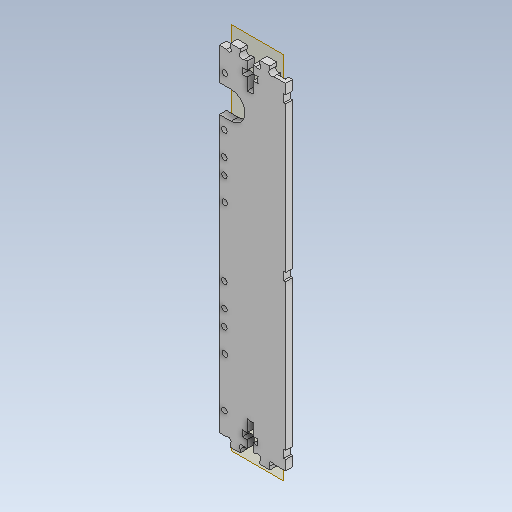
# Autodesk Inventor part: side_top
Saved by Autodesk Inventor 2020 (Build 240168000, 168)
## iProperties
Created: 2020-01-09
Part Number: side_top
Material: Generic
Document SubType Name: Modeling
Designer: erwin
Density: 1 g/cm^3
Appearance: Default
Author: erwin
Autodesk Inventor part; units mm, degrees
ref_plane "YZ Plane" through (0, 0, 0) normal (1, 0, 0) x (0, 1, 0)
ref_plane "XZ Plane" through (0, 0, 0) normal (0, 1, 0) x (-1, 0, 0)
ref_plane "XY Plane" through (0, 0, 0) normal (0, 0, 1) x (1, 0, 0)
ref_plane "Work Plane1" through (0, 0, 0) normal (0, 0, 1) x (1, 0, 0)
sketch "Sketch1" plane through (0, 0, 0) normal (0, 0, 1) x (1, 0, 0)
  line L0 (30, 0) -> (23.9528, 0) projected
  line L1 (30, 0) -> (30, -5) projected
  line L2 (23.9799, -170) -> (30, -170) projected
  line L3 (22, -171.9799) -> (22, -173.6) projected
  line L4 (22, -173.6) -> (17, -173.6) projected
  line L5 (17, -173.6) -> (17, -171.9799) projected
  line L6 (15.0201, -170) -> (13.5, -170) projected
  line L7 (13.5, -170) -> (13.5, -166) projected
  line L8 (13.5, -166) -> (16, -166) projected
  line L9 (16, -166) -> (16, -163) projected
  line L10 (16, -163) -> (13.5, -163) projected
  line L11 (13.5, -163) -> (13.5, -157) projected
  line L12 (13.5, -157) -> (10.5, -157) projected
  line L13 (10.5, -157) -> (10.5, -163) projected
  line L14 (10.5, -163) -> (8, -163) projected
  line L15 (8, -163) -> (8, -166) projected
  line L16 (8, -166) -> (10.5, -166) projected
  line L17 (10.5, -166) -> (10.5, -170) projected
  line L18 (10.5, -170) -> (8.9799, -170) projected
  line L19 (7, -171.9799) -> (7, -173.6) projected
  line L20 (7, -173.6) -> (2, -173.6) projected
  line L21 (2, -173.6) -> (2, -171.9799) projected
  line L22 (0.0201, -170) -> (-3.6, -170) projected
  line L23 (-3.6, -170) -> (-3.6, 0) projected
  line L24 (-3.6, 0) -> (0.0472, 0) projected
  line L25 (2, 1.9528) -> (2, 3.6) projected
  line L26 (2, 3.6) -> (7, 3.6) projected
  line L27 (7, 3.6) -> (7, 1.9799) projected
  line L28 (8.9799, 0) -> (10.5, 0) projected
  line L29 (10.5, 0) -> (10.5, -4) projected
  line L30 (10.5, -4) -> (8, -4) projected
  line L31 (8, -4) -> (8, -7) projected
  line L32 (8, -7) -> (10.5, -7) projected
  line L33 (10.5, -7) -> (10.5, -13) projected
  line L34 (10.5, -13) -> (13.5, -13) projected
  line L35 (13.5, -13) -> (13.5, -7) projected
  line L36 (13.5, -7) -> (16, -7) projected
  line L37 (16, -7) -> (16, -4) projected
  line L38 (16, -4) -> (13.5, -4) projected
  line L39 (13.5, -4) -> (13.5, 0) projected
  line L40 (13.5, 0) -> (15.0472, 0) projected
  line L41 (17, 1.9528) -> (17, 3.6) projected
  line L42 (17, 3.6) -> (22, 3.6) projected
  line L43 (22, 3.6) -> (22, 1.9528) projected
  line L44 (29, -165) -> (30, -165) projected
  line L45 (30, -5) -> (29, -5) projected
  line L46 (29, -5) -> (29, -9) projected
  line L47 (29, -9) -> (30, -9) projected
  line L48 (30, -9) -> (30, -83) projected
  line L49 (30, -83) -> (29, -83) projected
  line L50 (29, -83) -> (29, -87) projected
  line L51 (29, -87) -> (30, -87) projected
  line L52 (30, -87) -> (30, -161) projected
  line L53 (30, -161) -> (29, -161) projected
  line L54 (29, -161) -> (29, -165) projected
  arc A0 (17, -171.9799) -> (15.0201, -170) centre (16.0101, -170.9899) ccw projected
  arc A1 (8.9799, -170) -> (7, -171.9799) centre (7.9899, -170.9899) ccw projected
  arc A2 (2, -171.9799) -> (0.0201, -170) centre (1.0101, -170.9899) ccw projected
  arc A3 (0.0472, 0) -> (2, 1.9528) centre (1.1868, 0.8132) ccw projected
  arc A4 (7, 1.9799) -> (8.9799, 0) centre (7.9899, 0.9899) ccw projected
  arc A5 (15.0472, 0) -> (17, 1.9528) centre (16.1868, 0.8132) ccw projected
  arc A6 (22, 1.9528) -> (23.9528, 0) centre (22.8132, 0.8132) ccw projected
  line L55 (30, -165) -> (30, -170) projected
  arc A7 (23.9799, -170) -> (22, -171.9799) centre (22.9899, -170.9899) ccw projected
  circle A8 centre (-0.9899, -159.0101) radius 1.4 projected
  circle A9 centre (-0.8132, -134.0132) radius 1.4 projected
  circle A10 centre (-0.9899, -122.2101) radius 1.4 projected
  circle A11 centre (-0.9899, -114.1899) radius 1.4 projected
  circle A12 centre (-0.9899, -102.2101) radius 1.4 projected
  circle A13 centre (-0.8132, -67.6132) radius 1.4 projected
  circle A14 centre (-0.9899, -55.8101) radius 1.4 projected
  circle A15 centre (-0.9899, -47.7899) radius 1.4 projected
  circle A16 centre (-0.9899, -35.8101) radius 1.4 projected
  circle A17 centre (-0.8132, -10.8132) radius 1.4 projected
  point P0 (0, 0)
  point P1 (22, 0)
  point P2 (22, -170)
  point P3 (17, -170)
  point P4 (7, -170)
  point P5 (2, -170)
  point P6 (0, -160)
  point P7 (0, -123.2)
  point P8 (0, -113.2)
  point P9 (0, -103.2)
  point P10 (0, -56.8)
  point P11 (0, -46.8)
  point P12 (0, -36.8)
  point P13 (2, 0)
  point P14 (7, 0)
  point P15 (17, 0)
  point P16 (-1.9799, -160)
  point P17 (-1.9528, -133.2)
  point P18 (-1.9799, -123.2)
  point P19 (-1.9799, -113.2)
  point P20 (-1.9799, -103.2)
  point P21 (-1.9528, -66.8)
  point P22 (-1.9799, -56.8)
  point P23 (-1.9799, -46.8)
  point P24 (-1.9799, -36.8)
  point P25 (-1.9528, -10)
  point P26 (0, -34.8201)
  point P27 (0, -11.9528)
  point P28 (0, -54.8201)
  point P29 (0, -48.7799)
  point P30 (0, -101.2201)
  point P31 (0, -68.7528)
  point P32 (0, -121.2201)
  point P33 (0, -115.1799)
  point P34 (0, -158.0201)
  point P35 (0, -135.1528)
  constraints: 3 other
extrude "Extrusion1" add sketch "Sketch1" along normal blind 3.6
sketch "Sketch3" plane through (0, 0, 0) normal (0, 0, -1) x (-1, 0, 0)
  line L0 (-28, -170) -> (-24, -170) projected
  line L1 (-28, 0) -> (-28, -170) projected
  line L2 (-24, 0) -> (-28, 0) projected
  line L3 (-24, 0) -> (-24, -170) projected
  point P0 (0, 0)
extrude "Extrusion3" cut sketch "Sketch3" against normal blind 1.8
sketch "Sketch16" plane through (0, 0, 3.6) normal (0, 0, 1) x (1, 0, 0)
  line L0 (30, -87) -> (29, -87) projected
  line L1 (29, -87) -> (29, -83) projected
  line L2 (29, -83) -> (30, -83) projected
  line L3 (30, -83) -> (30, -9) projected
  line L4 (30, -9) -> (29, -9) projected
  line L5 (29, -9) -> (29, -5) projected
  line L6 (29, -5) -> (30, -5) projected
  line L7 (30, -5) -> (30, 0) projected
  line L8 (30, 0) -> (23.9528, 0) projected
  arc A0 (22, 1.9528) -> (23.9528, 0) centre (22.8132, 0.8132) ccw projected
  line L9 (22, 1.9528) -> (22, 3.6) projected
  line L10 (22, 3.6) -> (17, 3.6) projected
  line L11 (17, 3.6) -> (17, 1.9528) projected
  arc A1 (15.0472, 0) -> (17, 1.9528) centre (16.1868, 0.8132) ccw projected
  line L12 (15.0472, 0) -> (13.5, 0) projected
  line L13 (13.5, 0) -> (13.5, -4) projected
  line L14 (13.5, -4) -> (16, -4) projected
  line L15 (16, -4) -> (16, -7) projected
  line L16 (16, -7) -> (13.5, -7) projected
  line L17 (13.5, -7) -> (13.5, -13) projected
  line L18 (13.5, -13) -> (10.5, -13) projected
  line L19 (10.5, -13) -> (10.5, -7) projected
  line L20 (10.5, -7) -> (8, -7) projected
  line L21 (8, -7) -> (8, -4) projected
  line L22 (8, -4) -> (10.5, -4) projected
  line L23 (10.5, -4) -> (10.5, 0) projected
  line L24 (10.5, 0) -> (8.9799, 0) projected
  arc A2 (7, 1.9799) -> (8.9799, 0) centre (7.9899, 0.9899) ccw projected
  line L25 (7, 1.9799) -> (7, 3.6) projected
  line L26 (7, 3.6) -> (2, 3.6) projected
  line L27 (2, 3.6) -> (2, 1.9528) projected
  arc A3 (0.0472, 0) -> (2, 1.9528) centre (1.1868, 0.8132) ccw projected
  line L28 (0.0472, 0) -> (-3.6, 0) projected
  circle A4 centre (-0.8132, -10.8132) radius 1.4 projected
  circle A5 centre (-0.9899, -35.8101) radius 1.4 projected
  circle A6 centre (-0.9899, -47.7899) radius 1.4 projected
  circle A7 centre (-0.9899, -55.8101) radius 1.4 projected
  circle A8 centre (-0.8132, -67.6132) radius 1.4 projected
  circle A9 centre (-0.9899, -102.2101) radius 1.4 projected
  circle A10 centre (-0.9899, -114.1899) radius 1.4 projected
  circle A11 centre (-0.9899, -122.2101) radius 1.4 projected
  circle A12 centre (-0.8132, -134.0132) radius 1.4 projected
  circle A13 centre (-0.9899, -159.0101) radius 1.4 projected
  line L29 (-3.6, 0) -> (-3.6, -170) projected
  line L30 (-3.6, -170) -> (0.0201, -170) projected
  arc A14 (2, -171.9799) -> (0.0201, -170) centre (1.0101, -170.9899) ccw projected
  line L31 (2, -171.9799) -> (2, -173.6) projected
  line L32 (2, -173.6) -> (7, -173.6) projected
  line L33 (7, -173.6) -> (7, -171.9799) projected
  arc A15 (8.9799, -170) -> (7, -171.9799) centre (7.9899, -170.9899) ccw projected
  line L34 (8.9799, -170) -> (10.5, -170) projected
  line L35 (10.5, -170) -> (10.5, -166) projected
  line L36 (10.5, -166) -> (8, -166) projected
  line L37 (8, -166) -> (8, -163) projected
  line L38 (8, -163) -> (10.5, -163) projected
  line L39 (10.5, -163) -> (10.5, -157) projected
  line L40 (10.5, -157) -> (13.5, -157) projected
  line L41 (13.5, -157) -> (13.5, -163) projected
  line L42 (13.5, -163) -> (16, -163) projected
  line L43 (16, -163) -> (16, -166) projected
  line L44 (16, -166) -> (13.5, -166) projected
  line L45 (13.5, -166) -> (13.5, -170) projected
  line L46 (13.5, -170) -> (15.0201, -170) projected
  arc A16 (17, -171.9799) -> (15.0201, -170) centre (16.0101, -170.9899) ccw projected
  line L47 (17, -171.9799) -> (17, -173.6) projected
  line L48 (17, -173.6) -> (22, -173.6) projected
  line L49 (22, -173.6) -> (22, -171.9799) projected
  arc A17 (23.9799, -170) -> (22, -171.9799) centre (22.9899, -170.9899) ccw projected
  line L50 (23.9799, -170) -> (30, -170) projected
  line L51 (30, -170) -> (30, -165) projected
  line L52 (30, -165) -> (29, -165) projected
  line L53 (29, -165) -> (29, -161) projected
  line L54 (29, -161) -> (30, -161) projected
  line L55 (30, -161) -> (30, -87) projected
  line L56 (0, -30.4) -> (-3.6, -30.4) projected
  line L57 (0, -16.4) -> (-3.6, -16.4) projected
  line L58 (-3.6, -23.3865) -> (2.4, -23.3865) construction
  line L59 (-3.6, -16.3729) -> (2.4, -16.3729)
  line L60 (2.4, -30.4) -> (-3.6, -30.4)
  arc A18 (-3.6, -16.3729) -> (-3.6, -30.4) centre (-3.6, -23.3865) ccw
  arc A19 (2.4, -30.4) -> (2.4, -16.3729) centre (2.4, -23.3865) ccw
  point P0 (0, 0)
  point P1 (-0.6, -23.3865)
  dimension "d39" = 6
  constraints: 8 end point, 4 point on circle, 4 tangent, 2 centre point, 1 midpoint, 1 parallel
  measures "d39" distance of L58.start L58.end
extrude "Extrusion6" cut sketch "Sketch16" against normal through all contours A18 L29 | L29 L59 A19 L60 L56
sketch "Sketch17" plane through (0, 0, 3.6) normal (0, 0, 1) x (1, 0, 0)
  line L0 (-3.6, -16.3729) -> (2.4, -16.3729) projected
  arc A0 (2.4, -30.4) -> (2.4, -16.3729) centre (2.4, -23.3865) ccw projected
  line L1 (2.4, -30.4) -> (-3.6, -30.4) projected
  circle A1 centre (-0.9899, -35.8101) radius 1.4 projected
  circle A2 centre (-0.9899, -47.7899) radius 1.4 projected
  circle A3 centre (-0.9899, -55.8101) radius 1.4 projected
  circle A4 centre (-0.8132, -67.6132) radius 1.4 projected
  circle A5 centre (-0.9899, -102.2101) radius 1.4 projected
  circle A6 centre (-0.9899, -114.1899) radius 1.4 projected
  circle A7 centre (-0.9899, -122.2101) radius 1.4 projected
  circle A8 centre (-0.8132, -134.0132) radius 1.4 projected
  circle A9 centre (-0.9899, -159.0101) radius 1.4 projected
  line L2 (-3.6, 0) -> (-3.6, -16.3729) projected
  line L3 (-3.6, -170) -> (0.0201, -170) projected
  arc A10 (2, -171.9799) -> (0.0201, -170) centre (1.0101, -170.9899) ccw projected
  line L4 (2, -171.9799) -> (2, -173.6) projected
  line L5 (2, -173.6) -> (7, -173.6) projected
  line L6 (7, -173.6) -> (7, -171.9799) projected
  arc A11 (8.9799, -170) -> (7, -171.9799) centre (7.9899, -170.9899) ccw projected
  line L7 (8.9799, -170) -> (10.5, -170) projected
  line L8 (10.5, -170) -> (10.5, -166) projected
  line L9 (10.5, -166) -> (8, -166) projected
  line L10 (8, -166) -> (8, -163) projected
  line L11 (8, -163) -> (10.5, -163) projected
  line L12 (10.5, -163) -> (10.5, -157) projected
  line L13 (10.5, -157) -> (13.5, -157) projected
  line L14 (13.5, -157) -> (13.5, -163) projected
  line L15 (13.5, -163) -> (16, -163) projected
  line L16 (16, -163) -> (16, -166) projected
  line L17 (16, -166) -> (13.5, -166) projected
  line L18 (13.5, -166) -> (13.5, -170) projected
  line L19 (13.5, -170) -> (15.0201, -170) projected
  arc A12 (17, -171.9799) -> (15.0201, -170) centre (16.0101, -170.9899) ccw projected
  line L20 (17, -171.9799) -> (17, -173.6) projected
  line L21 (17, -173.6) -> (22, -173.6) projected
  line L22 (22, -173.6) -> (22, -171.9799) projected
  arc A13 (23.9799, -170) -> (22, -171.9799) centre (22.9899, -170.9899) ccw projected
  line L23 (23.9799, -170) -> (30, -170) projected
  line L24 (30, -170) -> (30, -165) projected
  line L25 (30, -165) -> (29, -165) projected
  line L26 (29, -165) -> (29, -161) projected
  line L27 (29, -161) -> (30, -161) projected
  line L28 (30, -161) -> (30, -87) projected
  line L29 (30, -87) -> (29, -87) projected
  line L30 (29, -87) -> (29, -83) projected
  line L31 (29, -83) -> (30, -83) projected
  line L32 (30, -83) -> (30, -9) projected
  line L33 (30, -9) -> (29, -9) projected
  line L34 (29, -9) -> (29, -5) projected
  line L35 (29, -5) -> (30, -5) projected
  line L36 (30, -5) -> (30, 0) projected
  line L37 (30, 0) -> (23.9528, 0) projected
  arc A14 (22, 1.9528) -> (23.9528, 0) centre (22.8132, 0.8132) ccw projected
  line L38 (22, 1.9528) -> (22, 3.6) projected
  line L39 (22, 3.6) -> (17, 3.6) projected
  line L40 (17, 3.6) -> (17, 1.9528) projected
  arc A15 (15.0472, 0) -> (17, 1.9528) centre (16.1868, 0.8132) ccw projected
  line L41 (15.0472, 0) -> (13.5, 0) projected
  line L42 (13.5, 0) -> (13.5, -4) projected
  line L43 (13.5, -4) -> (16, -4) projected
  line L44 (16, -4) -> (16, -7) projected
  line L45 (16, -7) -> (13.5, -7) projected
  line L46 (13.5, -7) -> (13.5, -13) projected
  line L47 (13.5, -13) -> (10.5, -13) projected
  line L48 (10.5, -13) -> (10.5, -7) projected
  line L49 (10.5, -7) -> (8, -7) projected
  line L50 (8, -7) -> (8, -4) projected
  line L51 (8, -4) -> (10.5, -4) projected
  line L52 (10.5, -4) -> (10.5, 0) projected
  line L53 (10.5, 0) -> (8.9799, 0) projected
  arc A16 (7, 1.9799) -> (8.9799, 0) centre (7.9899, 0.9899) ccw projected
  line L54 (7, 1.9799) -> (7, 3.6) projected
  line L55 (7, 3.6) -> (2, 3.6) projected
  line L56 (2, 3.6) -> (2, 1.9528) projected
  arc A17 (0.0472, 0) -> (2, 1.9528) centre (1.1868, 0.8132) ccw projected
  line L57 (0.0472, 0) -> (-3.6, 0) projected
  circle A18 centre (-0.8132, -10.8132) radius 1.4 projected
  line L58 (0, -153.6) -> (-3.6, -153.6) projected
  line L59 (0, -135.1528) -> (0, -158.0201) projected
  arc A19 (-0.2318, -139.5767) -> (5.2144, -151.2768) centre (0, -146.5865) ccw
  arc A20 (8.7055, -149.9855) -> (3.0039, -137.7368) centre (9.7399, -142.0526) ccw
  arc A21 (-0.2318, -139.5767) -> (3.0039, -137.7368) centre (-0.3641, -135.5789) ccw
  arc A22 (8.7055, -149.9855) -> (5.2144, -151.2768) centre (8.1883, -153.9519) ccw
  line L60 (-3.6, -30.4) -> (-3.6, -170) projected
  point P0 (0, 0)
  dimension "d42" = 16
  dimension "d43" = 4
  constraints: 9 point on circle, 4 centre point, 4 tangent, 1 equal radius, 1 midpoint
  measures "d42" diameter of A20
  measures "d43" radius of A21
extrude "Extrusion7" [suppressed]
equation "\"d0\" = wood_thickness"
equation "\"d7\" = deep_for_sliding_cover"
equation "\"wood_thickness\" = 3.6"
equation "\"deep_for_sliding_cover\" = 1.8"
body "Solid1"
